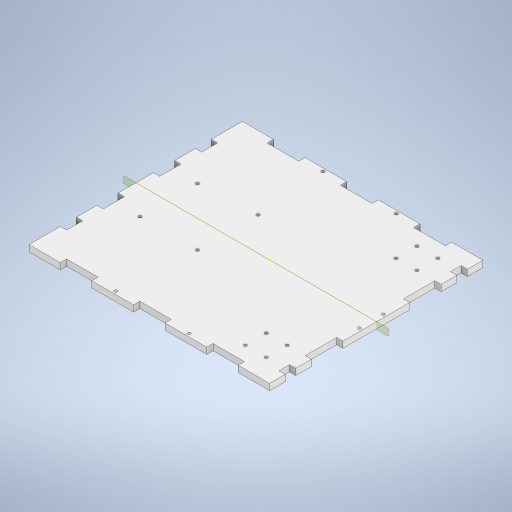
# Autodesk Inventor part: Низ робота
Saved by Autodesk Inventor 2024.2 (Build 282272000, 272)
## iProperties
Created: 2026-01-27
Part Number: Низ робота
Material: Типовые
Document SubType Name: Modeling
Designer: Service
Density: 1 g/cm^3
Appearance: Гладкий — белый
Author: Service
Autodesk Inventor part; units mm, degrees
ref_plane "YZ Plane" through (0, 0, 0) normal (1, 0, 0) x (0, 1, 0)
ref_plane "XZ Plane" through (0, 0, 0) normal (0, 1, 0) x (-1, 0, 0)
ref_plane "XY Plane" through (0, 0, 0) normal (0, 0, 1) x (1, 0, 0)
sketch "Эскиз1" plane through (0, 0, 0) normal (0, 1, 0) x (-1, 0, 0)
  line L0 (127.5386, 103.5005) -> (-102.4614, 103.5005)
  line L1 (-102.4614, 103.5005) -> (-102.4614, -100.4995)
  line L2 (-102.4614, -100.4995) -> (127.5386, -100.4995)
  line L3 (127.5386, -100.4995) -> (127.5386, 103.5005)
  line L4 (127.5386, -100.4995) -> (97.5386, -100.4995)
  line L5 (97.5386, -100.4995) -> (97.5386, -94.4995)
  line L6 (97.5386, -94.4995) -> (127.5386, -94.4995)
  line L7 (127.5386, -94.4995) -> (127.5386, -100.4995)
  line L8 (97.5386, -94.4995) -> (67.5386, -94.4995)
  line L9 (67.5386, -94.4995) -> (67.5386, -100.4995)
  line L10 (67.5386, -100.4995) -> (97.5386, -100.4995)
  line L11 (97.5386, -100.4995) -> (97.5386, -94.4995)
  line L12 (6.9803, -100.4995) -> (67.5386, -100.4995)
  line L13 (67.5386, -100.4995) -> (67.5386, -94.4995)
  line L14 (-42.4614, -94.4995) -> (-42.4614, -100.4995)
  line L15 (-42.4614, -100.4995) -> (-2.4614, -100.4995)
  line L16 (-42.4614, -94.4995) -> (-72.4614, -94.4995)
  line L17 (-72.4614, -94.4995) -> (-72.4614, -100.4995)
  line L18 (-72.4614, -100.4995) -> (-42.4614, -100.4995)
  line L19 (-42.4614, -100.4995) -> (-42.4614, -94.4995)
  line L20 (-72.4614, -94.4995) -> (-102.4614, -94.4995)
  line L21 (-102.4614, -94.4995) -> (-102.4614, -100.4995)
  line L22 (-102.4614, -100.4995) -> (-72.4614, -100.4995)
  line L23 (-72.4614, -100.4995) -> (-72.4614, -94.4995)
  line L24 (-42.4614, -94.4995) -> (-2.4614, -94.4995)
  line L25 (-2.4614, -94.4995) -> (-2.4614, -100.4995)
  line L26 (-2.4614, -100.4995) -> (-42.4614, -100.4995)
  line L27 (-42.4614, -100.4995) -> (-42.4614, -94.4995)
  line L28 (-2.4614, -100.4995) -> (27.5386, -100.4995)
  line L29 (27.5386, -100.4995) -> (27.5386, -94.4995)
  line L30 (27.5386, -94.4995) -> (-2.4614, -94.4995)
  line L31 (-2.4614, -94.4995) -> (-2.4614, -100.4995)
  line L32 (67.5386, -94.4995) -> (27.5386, -94.4995)
  line L33 (27.5386, -94.4995) -> (27.5386, -100.4995)
  line L34 (27.5386, -100.4995) -> (67.5386, -100.4995)
  line L35 (67.5386, -100.4995) -> (67.5386, -94.4995)
  line L36 (-102.4614, 97.5005) -> (127.5386, 97.5005)
  line L37 (127.5386, 97.5005) -> (97.5386, 97.5005)
  line L38 (97.5386, 97.5005) -> (97.5386, 103.5005)
  line L39 (97.5386, 103.5005) -> (127.5386, 103.5005)
  line L40 (127.5386, 103.5005) -> (127.5386, 97.5005)
  line L41 (97.5386, 103.5005) -> (67.5386, 103.5005)
  line L42 (67.5386, 103.5005) -> (67.5386, 97.5005)
  line L43 (67.5386, 97.5005) -> (97.5386, 97.5005)
  line L44 (97.5386, 97.5005) -> (97.5386, 103.5005)
  line L45 (6.9803, 97.5005) -> (67.5386, 97.5005)
  line L46 (67.5386, 97.5005) -> (67.5386, 103.5005)
  line L47 (-42.4614, 103.5005) -> (-42.4614, 97.5005)
  line L48 (-42.4614, 97.5005) -> (-2.4614, 97.5005)
  line L49 (-42.4614, 103.5005) -> (-72.4614, 103.5005)
  line L50 (-72.4614, 103.5005) -> (-72.4614, 97.5005)
  line L51 (-72.4614, 97.5005) -> (-42.4614, 97.5005)
  line L52 (-42.4614, 97.5005) -> (-42.4614, 103.5005)
  line L53 (-72.4614, 103.5005) -> (-102.4614, 103.5005)
  line L54 (-102.4614, 103.5005) -> (-102.4614, 97.5005)
  line L55 (-102.4614, 97.5005) -> (-72.4614, 97.5005)
  line L56 (-72.4614, 97.5005) -> (-72.4614, 103.5005)
  line L57 (-42.4614, 103.5005) -> (-2.4614, 103.5005)
  line L58 (-2.4614, 103.5005) -> (-2.4614, 97.5005)
  line L59 (-2.4614, 97.5005) -> (-42.4614, 97.5005)
  line L60 (-42.4614, 97.5005) -> (-42.4614, 103.5005)
  line L61 (-2.4614, 97.5005) -> (27.5386, 97.5005)
  line L62 (27.5386, 97.5005) -> (27.5386, 103.5005)
  line L63 (27.5386, 103.5005) -> (-2.4614, 103.5005)
  line L64 (-2.4614, 103.5005) -> (-2.4614, 97.5005)
  line L65 (67.5386, 103.5005) -> (27.5386, 103.5005)
  line L66 (27.5386, 103.5005) -> (27.5386, 97.5005)
  line L67 (27.5386, 97.5005) -> (67.5386, 97.5005)
  line L68 (67.5386, 97.5005) -> (67.5386, 103.5005)
  line L69 (-102.4614, 63.5005) -> (-96.4614, 63.5005)
  line L70 (-96.4614, 63.5005) -> (-96.4614, 33.5005)
  line L71 (-96.4614, 33.5005) -> (-102.4614, 33.5005)
  line L72 (-102.4614, 33.5005) -> (-102.4614, 63.5005)
  line L73 (-102.4614, -30.4995) -> (-96.4614, -30.4995)
  line L74 (-96.4614, -30.4995) -> (-96.4614, -60.4995)
  line L75 (-96.4614, -60.4995) -> (-102.4614, -60.4995)
  line L76 (-102.4614, -60.4995) -> (-102.4614, -30.4995)
  line L77 (127.5386, 63.5005) -> (121.5386, 63.5005)
  line L78 (121.5386, 33.5005) -> (127.5386, 33.5005)
  line L79 (127.5386, 33.5005) -> (127.5386, 63.5005)
  line L80 (127.5386, -50.4995) -> (93.2543, -50.4995)
  line L81 (121.5386, -60.4995) -> (127.5386, -60.4995)
  line L82 (127.5386, -60.4995) -> (127.5386, -50.4995)
  line L83 (-102.4614, 88.5005) -> (-96.4614, 88.5005)
  line L84 (-96.4614, 88.5005) -> (-96.4614, 78.5005)
  line L85 (-96.4614, 78.5005) -> (-102.4614, 78.5005)
  line L86 (-102.4614, 78.5005) -> (-102.4614, 88.5005)
  line L87 (-102.4614, -75.4995) -> (-96.4614, -75.4995)
  line L88 (-96.4614, -75.4995) -> (-96.4614, -85.4995)
  line L89 (-96.4614, -85.4995) -> (-102.4614, -85.4995)
  line L90 (-102.4614, -85.4995) -> (-102.4614, -75.4995)
  line L91 (127.5386, 73.5005) -> (121.5386, 73.5005)
  line L92 (121.5386, 73.5005) -> (121.5386, 58.5005)
  line L93 (121.5386, 58.5005) -> (127.5386, 58.5005)
  line L94 (127.5386, 58.5005) -> (127.5386, 73.5005)
  line L95 (127.5386, -55.4995) -> (121.5386, -55.4995)
  line L96 (121.5386, -55.4995) -> (121.5386, -70.4995)
  line L97 (121.5386, -70.4995) -> (127.5386, -70.4995)
  line L98 (127.5386, -70.4995) -> (127.5386, -55.4995)
  line L99 (127.5386, 38.5005) -> (121.5386, 38.5005)
  line L100 (121.5386, 38.5005) -> (121.5386, 18.5005)
  line L101 (121.5386, 18.5005) -> (127.5386, 18.5005)
  line L102 (127.5386, 18.5005) -> (127.5386, 38.5005)
  line L103 (127.5386, -15.4995) -> (121.5386, -15.4995)
  line L104 (121.5386, -15.4995) -> (121.5386, -35.4995)
  line L105 (121.5386, -35.4995) -> (127.5386, -35.4995)
  line L106 (127.5386, -35.4995) -> (127.5386, -15.4995)
  point P0 (0, 0)
  point P1 (-42.4614, -97.4995)
  point P2 (67.5386, -97.4995)
  point P3 (-42.4614, 100.5005)
  point P4 (67.5386, 100.5005)
  point P5 (-99.4614, -60.4995)
  point P6 (97.5386, 103.5005)
  point P7 (67.5386, 103.5005)
  point P8 (27.5386, 103.5005)
  point P9 (27.5386, 97.5005)
  point P10 (-2.4614, 103.5005)
  point P11 (-42.4614, 103.5005)
  point P12 (-102.4614, 33.5005)
  point P13 (-2.4614, -100.4995)
  point P14 (124.5386, 63.5005)
  point P15 (124.5386, -60.4995)
  point P16 (127.5386, 33.5005)
  point P17 (127.5386, 97.5005)
  point P18 (-102.4614, 97.5005)
  point P19 (97.5386, 97.5005)
  point P20 (27.5386, 103.5005)
  point P21 (-2.4614, 97.5005)
  point P22 (27.5386, 97.5005)
  point P23 (-2.4614, -100.4995)
  point P24 (-99.4614, 88.5005)
  point P25 (-99.4614, 78.5005)
  point P26 (-99.4614, 63.5005)
  point P27 (-99.4614, -75.4995)
  point P28 (124.5386, 73.5005)
  point P29 (124.5386, 58.5005)
  point P30 (124.5386, -70.4995)
  point P31 (124.5386, 38.5005)
  point P32 (124.5386, -55.4995)
  point P33 (124.5386, -35.4995)
  dimension "d0" = 230
  dimension "d1" = 204
  dimension "d2" = 6
  dimension "d3" = 30
  dimension "d4" = 30
  dimension "d5" = 30
  dimension "d6" = 30
  dimension "d8" = 40
  dimension "d10" = 40
  dimension "d11" = 230
  dimension "d13" = 6
  dimension "d14" = 30
  dimension "d15" = 30
  dimension "d16" = 30
  dimension "d17" = 30
  dimension "d18" = 40
  dimension "d19" = 40
  dimension "d20" = 40
  dimension "d21" = 30
  dimension "d22" = 40
  dimension "d23" = 30
  dimension "d24" = 6
  dimension "d27" = 6
  dimension "d28" = 40
  dimension "d29" = 40
  dimension "d30" = 30
  dimension "d31" = 30
  dimension "d84" = 10
  dimension "d85" = 15
  dimension "d86" = 15
  dimension "d87" = 10
  dimension "d88" = 6
  dimension "d89" = 6
  dimension "d90" = 15
  dimension "d91" = 15
  dimension "d92" = 30
  dimension "d93" = 30
  dimension "d94" = 20
  dimension "d95" = 20
  dimension "d96" = 20
  dimension "d97" = 20
  constraints: 214 end point, 48 parallel, 25 horizontal, 23 perpendicular, 21 point on line, 18 midpoint, 3 collinear
  measures "d0" distance of L1.end L2.end
  measures "d1" distance of L0.end L1.end
  measures "d2" distance of L4.end L5.end
  measures "d3" distance of L5.end L6.end
  measures "d4" distance of L16.end L20.end
  measures "d5" distance of L14.start L16.end
  measures "d6" distance of L5.end L8.end
  measures "d8" distance of L8.end L32.end
  measures "d10" distance of L14.start L24.end
  measures "d11" distance of L55.start L40.end
  measures "d13" distance of L38.start L41.start
  measures "d14" distance of L41.start L39.end
  measures "d15" distance of L53.start L53.end
  measures "d16" distance of L57.start L53.start
  measures "d17" distance of L41.start L42.start
  measures "d18" distance of L42.start L66.start
  measures "d19" distance of L57.start L57.end
  measures "d20" distance from line of point (-99.461, -60.5) L2
  measures "d21" distance of L73.end L74.end
  measures "d22" distance between parallel lines of L69 L0
  measures "d23" distance of L69.end L70.end
  measures "d24" distance of L70.end L71.end
  measures "d27" distance of L78.start L78.end
  measures "d28" distance from line of point (124.539, 63.5) L0
  measures "d29" distance from line of point (124.539, -60.5) L2
  measures "d30" distance of L80.end L81.start
  measures "d31" distance of L77.end L78.start
  measures "d84" distance of point (-99.461, 88.5) point (-99.461, 78.5)
  measures "d85" distance from line of point (-99.461, 63.5) L85
  measures "d86" distance from line of L75 point (-99.461, -75.5)
  measures "d87" distance of L87.end L88.end
  measures "d88" distance of L96.end L97.end
  measures "d89" distance of L92.end L93.end
  measures "d90" distance of point (124.539, 73.5) point (124.539, 58.5)
  measures "d91" distance of L95.end L96.end
  measures "d92" distance from line of L2 point (124.539, -70.5)
  measures "d93" distance from line of L0 point (124.539, 73.5)
  measures "d94" distance of L103.end L104.end
  measures "d95" distance of L99.end L100.end
  measures "d96" distance of point (124.539, 58.5) point (124.539, 38.5)
  measures "d97" distance of point (124.539, -55.5) point (124.539, -35.5)
extrude "Выдавливание1" add sketch "Эскиз1" along normal blind 6 contours L3 L36 L38 L0 | L3 L91 L92 L93 L99 L100 L101 L103 L104 L105 L95 L96 L97 L6 L8 L32 L30 L24 L16 L20 L1 L89 L88 L87 L75 L74 L73 L71 L70 L69 L85 L84 L83 L36 | L42 L36 L62 L0 | L58 L36 L47 L0 | L50 L36 L1 L0 | L3 L2 L5 L6 | L9 L2 L29 L32 | L20 L17 L2 L1 | L25 L2 L14 L24
sketch "Эскиз2" plane through (0, 6, 0) normal (0, 1, 0) x (1, 0, 0)
  point P0 (0, 0)
sketch "Эскиз5" plane through (0, 0, 0) normal (0, -1, 0) x (1, 0, 0)
  circle A0 centre (22.4614, 100.5005) radius 1.5
  circle A1 centre (-47.5386, 100.5005) radius 1.5
  circle A2 centre (-47.5386, -97.4995) radius 1.5
  circle A3 centre (22.4614, -97.4995) radius 1.5
  line L0 (42.4614, -100.4995) -> (2.4614, -100.4995) projected
  line L1 (-27.5386, -100.4995) -> (-67.5386, -100.4995) projected
  line L2 (42.4614, -94.4995) -> (42.4614, -100.4995) projected
  line L3 (-27.5386, -94.4995) -> (-27.5386, -100.4995) projected
  line L4 (2.4614, 103.5005) -> (42.4614, 103.5005) projected
  line L5 (-67.5386, 103.5005) -> (-27.5386, 103.5005) projected
  line L6 (2.4614, 97.5005) -> (2.4614, 103.5005) projected
  line L7 (-27.5386, 103.5005) -> (-27.5386, 97.5005) projected
  point P0 (0, 0)
  point P1 (42.4614, -97.4995)
  point P2 (2.4614, 100.5005)
  dimension "d41" = 3
  dimension "d42" = 3
  dimension "d43" = 3
  dimension "d44" = 20
  dimension "d45" = 20
  dimension "d46" = 3
  dimension "d47" = 3
  dimension "d48" = 20
  dimension "d49" = 20
  constraints: 4 centre point, 3 equal radius, 2 midpoint
  measures "d41" diameter of A3
  measures "d42" distance from line of L0 A3.centre
  measures "d43" distance from line of L1 A2.centre
  measures "d44" distance of point (42.461, -97.5) A3.centre
  measures "d45" distance from line of L3 A2.centre
  measures "d46" distance from line of L4 A0.centre
  measures "d47" distance from line of L5 A1.centre
  measures "d48" distance of A0.centre point (2.461, 100.5)
  measures "d49" distance from line of L7 A1.centre
extrude "Выдавливание3" cut sketch "Эскиз5" against normal through all
sketch "Эскиз6" plane through (0, 6, 0) normal (0, 1, 0) x (1, 0, 0)
  line L0 (76.6943, 94.4995) -> (62.6943, 94.4995) projected
  line L1 (62.2284, -103.5005) -> (76.2284, -103.5005) projected
  circle A0 centre (79.2284, -83.5005) radius 1.5
  circle A1 centre (59.2284, -83.5005) radius 1.5
  circle A2 centre (79.2284, -63.5005) radius 1.5
  circle A3 centre (59.2284, -63.5005) radius 1.5
  line L2 (79.2284, -159.6407) -> (79.2284, -82.1128) construction
  point P0 (0, 0)
  dimension "d52" = 3
  dimension "d53" = 20
  dimension "d54" = 20
  dimension "d55" = 20
  dimension "d56" = 20
  dimension "d57" = 20
  dimension "d58" = 20
  dimension "d59" = 3
  constraints: 4 centre point, 3 equal radius, 2 end point, 2 point on line, 1 vertical
  measures "d52" diameter of A0
  measures "d53" distance from line of L1 A0.centre
  measures "d54" distance from line of L1 A1.centre
  measures "d55" distance of A2.centre A3.centre
  measures "d56" distance of A2.centre A0.centre
  measures "d57" distance of A0.centre A1.centre
  measures "d58" distance of A3.centre A1.centre
  measures "d59" distance from line of L2 L1.end
extrude "Выдавливание4" cut sketch "Эскиз6" against normal through all
ref_plane "РабПлоскость1" through (42.4614, 0, 1.5005) normal (0, 0, -1) x (-1, 0, 0)
mirror "Зеркальное отражение1" about plane through (42.4614, 0, 1.5005) normal (0, 0, -1) of "Выдавливание4"
sketch "Эскиз7" plane through (0, 0, 0) normal (0, -1, 0) x (1, 0, 0)
  line L0 (96.4614, -60.4995) -> (96.4614, -30.4995)
  line L1 (96.4614, -30.4995) -> (102.4614, -30.4995)
  line L2 (102.4614, -30.4995) -> (102.4614, -60.4995)
  line L3 (102.4614, -60.4995) -> (96.4614, -60.4995)
  line L4 (96.4614, 39.5005) -> (96.4614, 69.5005)
  line L5 (96.4614, 69.5005) -> (102.4614, 69.5005)
  line L6 (102.4614, 69.5005) -> (102.4614, 33.5005)
  line L7 (102.4614, 39.5005) -> (96.4614, 39.5005)
  line L8 (102.4614, 13.4114) -> (96.4614, 13.4114) projected
  line L9 (96.4614, 16.4114) -> (102.4614, 16.4114) projected
  line L10 (96.4614, -6.5886) -> (102.4614, -6.5886) projected
  line L11 (102.4614, -9.5886) -> (96.4614, -9.5886) projected
  circle A0 centre (99.4614, 14.9114) radius 1.5
  circle A1 centre (99.4614, -8.0886) radius 1.5
  line L12 (102.4614, 33.5005) -> (102.4614, -30.4995) projected
  point P0 (0, 0)
  point P1 (99.4614, 13.4114)
  dimension "d62" = 3
  dimension "d63" = 3
  dimension "d64" = 3
  dimension "d65" = 3
  dimension "d66" = 1.5
  dimension "d67" = 1.5
  constraints: 16 end point, 4 horizontal, 4 vertical, 2 centre point, 1 midpoint, 8 other
  measures "d62" diameter of A1
  measures "d63" diameter of A0
  measures "d64" distance from line of L12 A1.centre
  measures "d65" distance from line of L12 A0.centre
  measures "d66" distance of point (99.461, 13.411) A0.centre
  measures "d67" distance from line of L10 A1.centre
extrude "Выдавливание5" cut sketch "Эскиз7" against normal blind 6 contours A0 | A1
sketch "Эскиз9" plane through (0, 0, 0) normal (0, -1, 0) x (1, 0, 0)
  circle A0 centre (-42.5386, 27.5005) radius 1.5
  circle A1 centre (-42.6205, -30.4995) radius 1.5
  circle A2 centre (-97.5386, -27.4995) radius 1.5
  circle A3 centre (-97.5386, 27.5005) radius 1.5
  line L0 (-127.5386, -100.4995) -> (-127.5386, 103.5005) projected
  line L1 (-97.5386, 97.5005) -> (-67.5386, 97.5005) projected
  line L2 (-27.5386, 97.5005) -> (2.4614, 97.5005) projected
  point P0 (0, 0)
  dimension "d70" = 3
  dimension "d71" = 3
  dimension "d72" = 3
  dimension "d73" = 3
  dimension "d74" = 55
  dimension "d75" = 52
  dimension "d76" = 55
  dimension "d77" = 52
  dimension "d78" = 30
  dimension "d79" = 30
  dimension "d80" = 70
  dimension "d81" = 70
  constraints: 4 centre point
  measures "d70" diameter of A1
  measures "d71" diameter of A2
  measures "d72" diameter of A3
  measures "d73" diameter of A0
  measures "d76" distance of A3.centre A2.centre
  measures "d78" distance from line of A3.centre L0
  measures "d79" distance from line of L0 A2.centre
  measures "d80" distance from line of L1 A3.centre
  measures "d81" distance from line of L2 A0.centre
extrude "Выдавливание6" cut sketch "Эскиз9" against normal up to surface (6 mm away)
